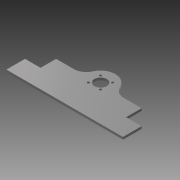
# Autodesk Inventor part: ZAxisNutMountMetal
Saved by Autodesk Inventor 2016 (Build 200138000, 138)
## iProperties
Category: Sheet Metal
Created: 2015-01-27
Part Number: ZAxisNutMountMetal
Material: Steel, Alloy
Document SubType Name: Modeling
Designer: Jack
Density: 7.73 g/cm^3
Appearance: Semi-Polished
Catalog Web Link: N/A
Mass: 35.5809 g
Surface Area: 143.094 cm^2
Volume: 35.5809 cm^3
Author: Jack
Title: Z Nut Mount
Autodesk Inventor part; units mm, degrees
ref_plane "YZ Plane" through (0, 0, 0) normal (1, 0, 0) x (0, 1, 0)
ref_plane "XZ Plane" through (0, 0, 0) normal (0, 1, 0) x (-1, 0, 0)
ref_plane "XY Plane" through (0, 0, 0) normal (0, 0, 1) x (1, 0, 0)
sketch "Sketch1" plane through (0, 0, 0) normal (0, 0, 1) x (1, 0, 0)
  line L0 (0, 0) -> (150, 0)
  line L1 (0, 0) -> (0, 24)
  line L2 (0, 24) -> (20, 24)
  circle A0 centre (75, 46.15) radius 8
  line L3 (20, 24) -> (20, 44)
  line L4 (20, 44) -> (56.122, 44)
  line L5 (150, 0) -> (150, 24)
  line L6 (150, 24) -> (130, 24)
  line L7 (130, 24) -> (130, 44)
  line L8 (130, 44) -> (93.878, 44)
  arc A1 (93.878, 44) -> (56.122, 44) centre (75, 46.15) ccw
  dimension "d0" = 150
  dimension "d1" = 24
  dimension "d3" = 16
  dimension "d4" = 20
  dimension "d5" = 38
  dimension "d6" = 75
  dimension "d7" = 22.15
  dimension "d19" = 20
  dimension "d20" = 20
  constraints: 18 end point, 4 perpendicular, 3 vertical, 2 centre point, 2 horizontal, 2 parallel, 2 point on circle, 1 coincident
  measures "d0" distance of L0.start L0.end
  measures "d1" distance of L0.start L1.end
  measures "d3" diameter of A0
  measures "d4" distance of L2.end L3.end
  measures "d5" diameter of A1
  measures "d6" distance from line of L5 A0.centre
  measures "d7" distance from line of A0.centre L6
  measures "d19" distance of L5.end L6.end
  measures "d20" distance of L1.end L2.end
extrude "Extrusion1" add sketch "Sketch1" along normal blind 3
fillet "Fillet1" radius 16 2 edges at (56.122, 44, 1.5) (93.878, 44, 1.5)
sketch "Sketch2" plane through (0, 0, 3) normal (0, 0, 1) x (1, 0, 0)
  circle A0 centre (82.7782, 53.9282) radius 1.5
  circle A1 centre (67.2218, 53.9282) radius 1.5
  circle A2 centre (67.2218, 38.3718) radius 1.5
  circle A3 centre (82.7782, 38.3718) radius 1.5
  circle A4 centre (75, 46.15) radius 8 projected
  circle A5 centre (75, 46.15) radius 11 construction
  line L0 (82.7782, 38.3718) -> (67.2218, 38.3718) construction
  line L1 (67.2218, 38.3718) -> (67.2218, 53.9282) construction
  dimension "d22" = 3
  dimension "d26" = 22
  constraints: 5 centre point, 4 end point, 4 point on circle, 3 equal radius, 2 horizontal alignment, 2 perpendicular, 2 vertical alignment, 1 coincident, 1 horizontal
  measures "d22" diameter of A3
  measures "d26" diameter of A5
extrude "Extrusion2" cut sketch "Sketch2" against normal up to surface (3 mm away) contours A0 | A1 | A2 | A3
sketch "Sketch3" plane through (0, 0, 3) normal (0, 0, 1) x (1, 0, 0)
  line L0 (0, 0) -> (150, 0) projected
  line L1 (150, 0) -> (150, 24) projected
  line L2 (0, 24) -> (0, 0) projected
  point P0 (10, 12)
  point P1 (140, 12)
  dimension "d27" = 10
  dimension "d28" = 10
  dimension "d29" = 12
  constraints: 1 horizontal alignment
  measures "d27" distance from line of L2 point (10, 12)
  measures "d28" distance from line of L1 point (140, 12)
  measures "d29" distance from line of L0 point (140, 12)
hole "Hole1" at (10, 12, 3) at (140, 12, 3) direction (0, 0, -1) diameter 5 end through all
body "Solid1"
